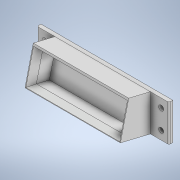
# Autodesk Inventor part: FlaskHolderTilted_13_1_final
Saved by Autodesk Inventor 2020 (Build 240168000, 168)
## iProperties
Created: 2023-03-07
Part Number: FlaskHolderTilted_13_1_final
Material: Generic
Document SubType Name: Modeling
Designer: DSOB
Density: 1 g/cm^3
Appearance: Default
Author: DSOB
Autodesk Inventor part; units mm, degrees
ref_plane "YZ Plane" through (0, 0, 0) normal (1, 0, 0) x (0, 1, 0)
ref_plane "XZ Plane" through (0, 0, 0) normal (0, 1, 0) x (-1, 0, 0)
ref_plane "XY Plane" through (0, 0, 0) normal (0, 0, 1) x (1, 0, 0)
sketch "Sketch1" plane through (0, 0, 0) normal (0, 0, 1) x (1, 0, 0)
  line L0 (0, 0) -> (170, 0)
  line L1 (170, 0) -> (170, 47.1)
  line L2 (170, 47.1) -> (0, 47.1)
  line L3 (0, 47.1) -> (0, 0)
  dimension "d0" = 170
  dimension "d1" = 47.1
  constraints: 8 end point, 2 parallel, 1 horizontal, 1 perpendicular
  measures "d0" distance of L1.end L2.end
  measures "d1" distance of L0.end L1.end
extrude "Extrusion1" add sketch "Sketch1" along normal blind 5
sketch "Sketch2" plane through (0, 0, 5) normal (0, 0, 1) x (1, 0, 0)
  line L0 (0, 0) -> (170, 0) projected
  line L1 (170, 47.1) -> (0, 47.1) projected
  line L2 (146, 0) -> (23, 0)
  line L3 (23, 0) -> (23, 47.1)
  line L4 (23, 47.1) -> (146, 47.1)
  line L5 (146, 47.1) -> (146, 0)
  line L6 (143, 2.8) -> (26, 2.8)
  line L7 (26, 2.8) -> (26, 44.3)
  line L8 (26, 44.3) -> (143, 44.3)
  line L9 (143, 44.3) -> (143, 2.8)
  line L10 (170, 0) -> (170, 47.1) projected
  point P0 (146, 47.1)
  point P1 (23, 0)
  dimension "d4" = 123
  dimension "d5" = 117
  dimension "d6" = 3
  dimension "d7" = 2.8
  dimension "d8" = 2.8
  dimension "d9" = 24
  constraints: 16 end point, 4 parallel, 2 horizontal, 2 perpendicular, 2 point on line
  measures "d4" distance between parallel lines of L3 L5
  measures "d5" distance of L6.start L6.end
  measures "d6" distance between parallel lines of L3 L7
  measures "d7" distance between parallel lines of L0 L6
  measures "d8" distance between parallel lines of L1 L8
  measures "d9" distance between parallel lines of L5 L10
sketch "Sketch3" plane through (0, 0, 5) normal (0, 0, 1) x (1, 0, 0)
  circle A0 centre (160, 11) radius 3.25
  circle A1 centre (160, 36) radius 3.25
  line L0 (170, 0) -> (170, 47.1) projected
  line L1 (0, 0) -> (170, 0) projected
  line L2 (85, -16.6248) -> (85, 70.7208)
  line L3 (0, 47.1) -> (0, 0) projected
  circle A2 centre (10, 11) radius 3.25
  circle A3 centre (10, 36) radius 3.25
  point P0 (146, 0)
  dimension "d21" = 6.5
  dimension "d22" = 6.5
  dimension "d23" = 10
  dimension "d24" = 10
  dimension "d25" = 25
  dimension "d26" = 11
  dimension "d27" = 85
  constraints: 4 centre point, 2 end point, 2 symmetric about line, 1 vertical, 2 other
  measures "d21" diameter of A0
  measures "d22" diameter of A1
  measures "d23" distance from line of L0 A0.centre
  measures "d24" distance from line of L0 A1.centre
  measures "d25" distance of A0.centre A1.centre
  measures "d26" distance from line of L1 A0.centre
  measures "d27" distance between parallel lines of L3 L2
extrude "Extrusion3" cut sketch "Sketch3" against normal blind 60
sketch "Sketch4" plane through (0, 0, 0) normal (-1, 0, 0) x (0, 0, 1)
  line L0 (5, 0) -> (5, 47) projected
  line L1 (5, 23.5) -> (58.7, 36.3922)
  point P0 (0, 0)
  dimension "d30" = 76.5
  constraints: 2 end point, 1 midpoint
  measures "d30" angle of L0 L1
sweep "Sweep1" add profiles "Sketch2" path "Sketch4" separate body path curves L1 contours L3 L1 L5 L0
sketch "Sketch5" plane through (23, 0, 5) normal (-1, 0, 0) x (0, 0, 1)
  line L0 (0, 47.1) -> (53.7, 59.9922) projected
  line L1 (0, 47.1) -> (10.6915, 2.5668)
  line L2 (0, 0) -> (53.7, 12.8922) projected
  line L3 (0, 47.1) -> (0, 0) projected
  line L4 (0, 0) -> (0, 47.1)
  point P0 (-5, 0)
  dimension "d42" = 13.5
  constraints: 4 end point, 1 collinear, 1 point on line
  measures "d42" angle of L3 L1
extrude "Extrusion4" add sketch "Sketch5" against normal up to surface (123 mm away) bodies 2
sketch "Sketch6" plane through (23, 0, 5) normal (-1, 0, 0) x (0, 0, 1)
  line L0 (0, 0) -> (53.7, 12.8922) projected
  line L1 (53.7, 59.9922) -> (53.7, 12.8922)
  line L2 (0, 47.1) -> (53.7, 59.9922) projected
  line L3 (53.7, 59.9922) -> (27.8412, 53.7841)
  line L4 (27.8412, 53.7841) -> (38.5327, 9.2509)
  line L5 (0, 0) -> (53.7, 12.8922) projected
  line L6 (38.5327, 9.2509) -> (53.7, 12.8922)
  point P0 (-5, 0)
  point P1 (38.5327, 9.2509)
  dimension "d59" = 13.5
  constraints: 8 end point, 2 point on line, 1 parallel, 1 vertical
  measures "d59" angle of L1 L4
extrude "Extrusion5" cut sketch "Sketch6" against normal through all bodies 2
fillet "Fillet3" radius 2 2 edges at (0, 23.55, 5) (170, 23.55, 5)
chamfer "Chamfer11" distance 2 angle 80 1 edges at (84.5, 11.8983, 42.8971) measured on face at (65, 10.1333, 43.3208)
chamfer "Chamfer12" distance 2 angle 80 1 edges at (143, 31.5175, 38.1869) measured on face at (104, 52.9016, 33.0531)
chamfer "Chamfer13" distance 2 angle 80 1 edges at (26, 31.5175, 38.1869) measured on face at (104, 52.9016, 33.0531)
body "Solid1"
body "Solid2"
